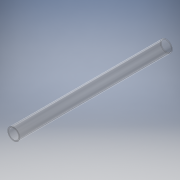
# Autodesk Inventor part: Tubo33mmx50cm
Saved by Autodesk Inventor 2017 (Build 210142000, 142)
## iProperties
Part Number: Tubo33mmx50cm
Material: Policarbonato, claro
Document SubType Name: Modeling
Designer: Leonardo
Density: 1.2 g/cm^3
Appearance: Policarbonato - Claro
Author: Leonardo
Autodesk Inventor part; units mm, degrees
ref_plane "YZ Plane" through (0, 0, 0) normal (1, 0, 0) x (0, 1, 0)
ref_plane "XZ Plane" through (0, 0, 0) normal (0, 1, 0) x (-1, 0, 0)
ref_plane "XY Plane" through (0, 0, 0) normal (0, 0, 1) x (1, 0, 0)
sketch "Boceto1" plane through (0, 0, 0) normal (0, 1, 0) x (-1, 0, 0)
  circle A0 centre (0, 0) radius 16.5
  circle A1 centre (0, 0) radius 19.85
  dimension "d0" = 33
  dimension "d1" = 39.7
  constraints: 2 centre point, 2 coincident
  measures "d0" diameter of A0
  measures "d1" diameter of A1
extrude "Extrusión1" add sketch "Boceto1" along normal blind 500
